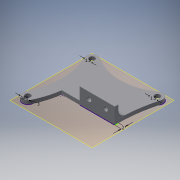
# Autodesk Inventor part: FanMount
Saved by Autodesk Inventor 2018 (Build 220112000, 112)
## iProperties
Created: 2020-01-21
Part Number: FanMount
Material: Generic
Document SubType Name: Modeling
Designer: Vinnie Caprarola
Density: 1 g/cm^3
Appearance: Default
Author: Vinnie Caprarola
Autodesk Inventor part; units mm, degrees
ref_plane "YZ Plane" through (0, 0, 0) normal (1, 0, 0) x (0, 1, 0)
ref_plane "XZ Plane" through (0, 0, 0) normal (0, 1, 0) x (-1, 0, 0)
ref_plane "Work Plane1" through (0, 0, 0) normal (0, 0, 1) x (1, 0, 0)
sketch "Sketch2" plane through (0, 0, 0) normal (0, 0, 1) x (1, 0, 0)
  circle A0 centre (-17.6777, 17.6777) radius 3 projected
  circle A1 centre (17.6777, 17.6777) radius 3 projected
  circle A2 centre (-17.6777, -17.1777) radius 3 projected
  line L0 (17.7, -5.427) -> (-1.3, -5.427) projected
  line L1 (-1.3, -5.427) -> (17.7, -5.427)
  line L2 (17.7, -5.427) -> (17.7, -3.927)
  line L3 (17.7, -3.927) -> (-1.3, -3.927)
  line L4 (-1.3, -3.927) -> (-1.3, -5.427)
  arc A3 (-15.9573, 20.1354) -> (15.9573, 20.1354) centre (0, 42.9323) ccw
  arc A4 (-20.3689, -15.8521) -> (-20.3689, 16.3521) centre (-53.0613, 0.25) ccw
  arc A5 (-14.9864, -18.5032) -> (-11, -5.427) centre (-53.0613, 0.25) ccw
  line L5 (-11, -5.427) -> (-1.3, -5.427)
  arc A6 (20.5658, 16.8661) -> (17.7, -3.927) centre (94.5659, -3.927) ccw
  circle A7 centre (-17.6777, 17.6777) radius 1.5
  circle A8 centre (17.6777, 17.6777) radius 1.5
  circle A9 centre (-17.6777, -17.1777) radius 1.5
  point P0 (0, 0)
  point P1 (-10.5, -5.427)
  dimension "d6" = 19
  dimension "d7" = 1.5
  dimension "d9" = 0.5
  dimension "d10" = 3
  dimension "d11" = 3
  dimension "d12" = 3
  constraints: 14 point on circle, 10 end point, 7 centre point, 7 tangent, 3 coincident, 2 parallel, 1 collinear, 1 concentric, 1 horizontal, 1 horizontal alignment, 1 perpendicular, 1 other
  measures "d6" distance of L3.end L2.end
  measures "d7" distance of L2.end L1.end
  measures "d9" distance of point (-10.5, -5.427) L5.start
  measures "d10" diameter of A7
  measures "d11" diameter of A8
  measures "d12" diameter of A9
extrude "Extrusion1" add sketch "Sketch2" along normal blind 2
sketch "Sketch3" plane through (0, 0, 2) normal (0, 0, 1) x (1, 0, 0)
  line L0 (-11, -5.427) -> (17.7, -5.427) projected
  line L1 (17.7, -5.427) -> (-1.3, -5.427)
  line L2 (-1.3, -5.427) -> (-1.3, -3.427)
  line L3 (-1.3, -3.427) -> (17.7, -3.427)
  line L4 (17.7, -3.427) -> (17.7, -5.427)
  point P0 (0, 0)
  dimension "d15" = 19
  dimension "d16" = 2
  constraints: 8 end point, 2 parallel, 1 horizontal, 1 perpendicular
  measures "d15" distance of L2.end L3.end
  measures "d16" distance of L1.end L2.end
ref_plane "Work Plane2" through (-1.3, -10.427, 8.7) normal (0, 0, 1) x (1, 0, 0)
extrude "Extrusion2" add sketch "Sketch3" along normal up to surface (6.7 mm away)
sketch "Sketch4" plane through (-1.3, -3.427, 2) normal (0, 1, 0) x (1, 0, 0)
  circle A0 centre (14, -3.2) radius 1.25 projected
  circle A1 centre (5, -3.2) radius 1.25 projected
  circle A2 centre (5, -3.2) radius 3
  circle A3 centre (14, -3.2) radius 3
  point P0 (1.3, 2)
  dimension "d20" = 6
  dimension "d21" = 6
  constraints: 2 centre point, 2 coincident
  measures "d20" diameter of A2
  measures "d21" diameter of A3
fillet "Fillet1" radius 4 1 edges at (8.2, -3.427, 2)
extrude "Extrusion3" cut sketch "Sketch4" along normal blind 10 contours A0 | A1 | A2 | A3
hole "Hole1" at (3.7, -3.427, 5.2) direction (0, -1, 0) diameter 2.5 end through all
hole "Hole2" at (12.7, -3.427, 5.2) direction (0, -1, 0) diameter 2.5 end through all
body "Solid1"
